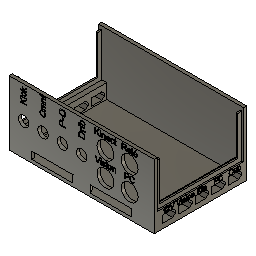
BlackBox+v3 (Autodesk Fusion 360 design; units mm, degrees)
Autodesk Fusion 360 part; units mm, degrees
(part 1 of 2)
sketch "Esboço1" plane through (0, 0, 0) normal (0, 1, 0) x (1, 0, 0)
  line L0 (0, 0) -> (0, -40)
  line L1 (90, 0) -> (-90, 0)
  line L2 (-90, 0) -> (-90, -80)
  line L3 (-90, -80) -> (90, -80)
  line L4 (90, -80) -> (90, 0)
  line L5 (90, 0) -> (-90, -80) construction
  line L6 (-90, 0) -> (90, -80) construction
  line L7 (90, -80) -> (70, -80)
  line L8 (70, -80) -> (70, -70)
  line L9 (70, -70) -> (90, -70)
  line L10 (90, -70) -> (90, -80)
  line L11 (70, -70) -> (49, -70)
  line L12 (49, -70) -> (49, -49)
  line L13 (49, -49) -> (70, -49)
  line L14 (70, -49) -> (70, -70)
  circle A0 centre (59.5, -59.5) radius 10.5
  circle A1 centre (29.5, -59.5) radius 10.5
  circle A2 centre (59.5, -29.5) radius 10.5
  circle A3 centre (29.5, -29.5) radius 10.5
  circle A4 centre (0, -40) radius 6.5
  line L15 (7.5, -24.75) -> (-7.5, -24.75)
  line L16 (-7.5, -24.75) -> (-7.5, -55.25)
  line L17 (-7.5, -55.25) -> (7.5, -55.25)
  line L18 (7.5, -55.25) -> (7.5, -24.75)
  line L19 (7.5, -24.75) -> (-7.5, -55.25) construction
  line L20 (-7.5, -24.75) -> (7.5, -55.25) construction
  line L21 (-31.5, -24.75) -> (-31.5, -55.25)
  line L22 (-31.5, -24.75) -> (-16.5, -55.25) construction
  line L23 (-16.5, -24.75) -> (-31.5, -55.25) construction
  line L24 (-31.5, -55.25) -> (-16.5, -55.25)
  circle A5 centre (-24, -40) radius 6.5
  line L25 (-16.5, -24.75) -> (-31.5, -24.75)
  line L26 (-16.5, -55.25) -> (-16.5, -24.75)
  line L27 (-55.5, -24.75) -> (-55.5, -55.25)
  line L28 (-55.5, -24.75) -> (-40.5, -55.25) construction
  line L29 (-40.5, -24.75) -> (-55.5, -55.25) construction
  line L30 (-55.5, -55.25) -> (-40.5, -55.25)
  circle A6 centre (-48, -40) radius 6.5
  line L31 (-40.5, -24.75) -> (-55.5, -24.75)
  line L32 (-40.5, -55.25) -> (-40.5, -24.75)
  line L33 (-79.5, -24.75) -> (-79.5, -55.25)
  line L34 (-79.5, -24.75) -> (-64.5, -55.25) construction
  line L35 (-64.5, -24.75) -> (-79.5, -55.25) construction
  line L36 (-79.5, -55.25) -> (-64.5, -55.25)
  circle A7 centre (-72, -40) radius 6.5
  line L37 (-64.5, -24.75) -> (-79.5, -24.75)
  line L38 (-64.5, -55.25) -> (-64.5, -24.75)
  line L39 (-86, -80) -> (-86, -4)
  line L40 (90, -80) -> (86, -80)
  line L41 (86, -80) -> (86, -4)
  line L42 (86, -4) -> (-86, -4)
  line L43 (11.25, -4) -> (11.25, -80)
  line L44 (15.25, -80) -> (15.25, -4)
  line L45 (15.25, -4) -> (11.25, -80) construction
  line L46 (11.25, -4) -> (15.25, -80) construction
  line L47 (-86, -4) -> (-62, -4)
  line L48 (-62, -4) -> (-7, -4)
  line L49 (-7, -4) -> (-7, -13)
  line L50 (-7, -13) -> (-62, -13)
  line L51 (-62, -13) -> (-62, -4)
  line L52 (86, -4) -> (62, -4)
  line L53 (62, -4) -> (7, -4)
  line L54 (7, -4) -> (7, -13)
  line L55 (7, -13) -> (62, -13)
  line L56 (62, -13) -> (62, -4)
  line L57 (86, -4) -> (86, -22)
  line L58 (86, -22) -> (90, -22)
  line L59 (-86, -4) -> (-86, -22)
  line L60 (-86, -22) -> (-90, -22)
  line L61 (-86, -4) -> (-90, -4)
  line L62 (86, -4) -> (90, -4)
  line L63 (29.5, -40) -> (29.5, -49)
  line L64 (39.5, -48.5) -> (19.5, -48.5)
  line L65 (19.5, -48.5) -> (19.5, -40.5)
  line L66 (19.5, -40.5) -> (39.5, -40.5)
  line L67 (39.5, -40.5) -> (39.5, -48.5)
  line L68 (39.5, -48.5) -> (19.5, -40.5) construction
  line L69 (19.5, -48.5) -> (39.5, -40.5) construction
  line L70 (19.5, -40.5) -> (39.5, -40.5) construction
  line L71 (39.5, -40.5) -> (39.5, -48.5) construction
  line L72 (39.5, -48.5) -> (19.5, -48.5) construction
  line L73 (19.5, -48.5) -> (19.5, -40.5) construction
  line L74 (19.5, -70.5) -> (39.5, -70.5) construction
  line L75 (39.5, -70.5) -> (39.5, -78.5) construction
  line L76 (39.5, -78.5) -> (19.5, -78.5) construction
  line L77 (19.5, -78.5) -> (19.5, -70.5) construction
  line L78 (49.5, -40.5) -> (69.5, -40.5) construction
  line L79 (69.5, -40.5) -> (69.5, -48.5) construction
  line L80 (69.5, -48.5) -> (49.5, -48.5) construction
  line L81 (49.5, -48.5) -> (49.5, -40.5) construction
  line L82 (49.5, -70.5) -> (69.5, -70.5) construction
  line L83 (69.5, -70.5) -> (69.5, -78.5) construction
  line L84 (69.5, -78.5) -> (49.5, -78.5) construction
  line L85 (49.5, -78.5) -> (49.5, -70.5) construction
  line L86 (4.0716, -57.4789) -> (4.0716, -77.4789) construction
  line L87 (4.0716, -77.4789) -> (-3.9284, -77.4789) construction
  line L88 (-3.9284, -77.4789) -> (-3.9284, -57.4789) construction
  line L89 (-3.9284, -57.4789) -> (4.0716, -57.4789) construction
  line L90 (-20.0052, -57.4897) -> (-20.0052, -77.4897) construction
  line L91 (-20.0052, -77.4897) -> (-28.0052, -77.4897) construction
  line L92 (-28.0052, -77.4897) -> (-28.0052, -57.4897) construction
  line L93 (-28.0052, -57.4897) -> (-20.0052, -57.4897) construction
  line L94 (-68.5263, -57.4789) -> (-68.5263, -77.4789) construction
  line L95 (-68.5263, -77.4789) -> (-76.5263, -77.4789) construction
  line L96 (-76.5263, -77.4789) -> (-76.5263, -57.4789) construction
  line L97 (-76.5263, -57.4789) -> (-68.5263, -57.4789) construction
  line L98 (-44.4564, -57.7899) -> (-44.5481, -77.8423) construction
  line L99 (-44.5481, -77.8423) -> (-52.4163, -77.8063) construction
  line L100 (-52.4163, -77.8063) -> (-52.3246, -57.7539) construction
  line L101 (-52.3246, -57.7539) -> (-44.4564, -57.7899) construction
  point P0 (0, -40)
  point P1 (0, -40)
  point P2 (-24, -40)
  point P3 (-24, -40)
  point P4 (-24, -40)
  point P5 (-48, -40)
  point P6 (-48, -40)
  point P7 (-48, -40)
  point P8 (-72, -40)
  point P9 (-72, -40)
  point P10 (-72, -40)
  point P11 (13.25, -42)
  point P12 (29.5, -44.5)
  dimension "d1" = 40
  dimension "d2" = 180
  dimension "d3" = 80
  dimension "d4" = 20
  dimension "d5" = 10
  dimension "d6" = 21
  dimension "d7" = 21
  dimension "d10" = -30
  dimension "d11" = 30
  dimension "d12" = 13
  dimension "d13" = 15
  dimension "d14" = 30.5
  dimension "d17" = -24
  dimension "d18" = 0
  dimension "d19" = 4
  dimension "d21" = 4
  dimension "d23" = 4
  dimension "d33" = 24
  dimension "d34" = 55
  dimension "d35" = 9
  dimension "d36" = 24
  dimension "d37" = 55
  dimension "d38" = 9
  dimension "d72" = 18
  dimension "d73" = 18
  dimension "d124" = 20
  dimension "d125" = 8
  dimension "d126" = 7
  dimension "d127" = 7
  dimension "d128" = 7
  dimension "d129" = 7
  dimension "d130" = 8
  dimension "d131" = 8
  dimension "d132" = 7
  dimension "d133" = 7
  text T0 "Vision" font "Arial" height 7 align centre middle in box 20 x 8 at (19.5, -40.5) x (1, 0) y (0, -1) spacing 1 kerned
  text T1 "Kinect" font "Arial" height 7 align centre middle in box 20 x 8 at (19.5, -70.5) x (1, 0) y (0, -1) spacing 1 kerned
  text T2 "PC" font "Arial" height 7 align centre middle in box 20 x 8 at (49.5, -40.5) x (1, 0) y (0, -1) spacing 1 kerned
  text T3 "Relé" font "Arial" height 7 align centre middle in box 20 x 8 at (49.5, -70.5) x (1, 0) y (0, -1) spacing 1 kerned
  text T4 "Drib" font "Arial" height 8 align centre middle in box 20 x 8 at (4.0716, -57.4789) x (0, -1) y (-1, 0) spacing 1 kerned
  text T5 "P-O" font "Arial" height 8 align centre middle in box 20 x 8 at (-20.0052, -57.4897) x (0, -1) y (-1, 0) spacing 1 kerned
  text T6 "Kick" font "Arial" height 7 align centre middle in box 20 x 8 at (-68.5263, -57.4789) x (0, -1) y (-1, 0) spacing 1 kerned
  text T7 "Omni" font "Arial" height 7 align centre middle in box 20.0526 x 7.8682 at (-44.4564, -57.7899) x (-0.004573, -0.99999) y (-0.99999, 0.004573) spacing 1 kerned
  constraint coincident L0.start origin
  constraint vertical L0
  constraint horizontal L1
  constraint parallel L2 L4
  constraint coincident L5 P1
  constraint coincident L6 P1
  constraint coincident P1 P0
  constraint horizontal L7
  constraint vertical L8
  constraint horizontal L9
  constraint vertical L10
  constraint horizontal L11
  constraint vertical L12
  constraint horizontal L13
  constraint vertical L14
  constraint tangent L11 A0
  constraint tangent L14 A0
  constraint tangent L13 A0
  constraint horizontal L15
  constraint perpendicular L15 L16
  constraint parallel L15 L17
  constraint parallel L16 L18
  constraint coincident L19 P1
  constraint coincident L20 P1
  constraint coincident L3 L39.start
  constraint coincident L7 L40.end
  constraint parallel L43 L44
  constraint coincident L45 P11
  constraint coincident L46 P11
  constraint coincident L42 L47.end
  constraint perpendicular L39 L47
  constraint horizontal L48
  constraint vertical L49
  constraint horizontal L50
  constraint vertical L51
  constraint coincident L42 L52.end
  constraint perpendicular L41 L52
  constraint horizontal L53
  constraint vertical L54
  constraint horizontal L55
  constraint vertical L56
  constraint coincident L41 L57.end
  constraint coincident L4 L58.end
  constraint perpendicular L4 L58
  constraint coincident L39 L59.end
  constraint coincident L2 L60.end
  constraint perpendicular L2 L60
  constraint coincident L2 L61.end
  constraint perpendicular L2 L61
  constraint coincident L4 L62.end
  constraint perpendicular L4 L62
  constraint coincident A3 L63.start
  constraint coincident A1 L63.end
  constraint vertical L63
  constraint horizontal L64
  constraint perpendicular L64 L65
  constraint parallel L64 L66
  constraint parallel L65 L67
  constraint coincident L68 P12
  constraint coincident L69 P12
  constraint midpoint L63 P12
  constraint coincident L66.end
  constraint coincident L64.end
  measures "d1" distance of L0.start P0
  measures "d2" distance of L2.end L3.end
  measures "d3" distance of L1.end L2.end
  measures "d4" distance of L3.end L7.end
  measures "d5" distance of L3.end L9.end
  measures "d6" distance of L8.end L11.end
  measures "d7" distance of L8.end L13.end
  measures "d12" diameter of A4
  measures "d13" distance of L16.end L17.end
  measures "d14" distance of L15.end L16.end
  measures "d19" distance of L2.end L39.start
  measures "d21" distance of L3.end L40.end
  measures "d23" distance of L43.end L44.start
  measures "d33" distance of L39.end L47.end
  measures "d34" distance of L47.end L48.end
  measures "d35" distance of L47.end L50.end
  measures "d36" distance of L41.end L52.end
  measures "d37" distance of L52.end L53.end
  measures "d38" distance of L52.end L55.end
  measures "d72" distance of L41.end L57.end
  measures "d73" distance of L39.end L59.end
  measures "d124" distance of L65.end L66.end
  measures "d125" distance of L64.end L65.end
sketch "Esboço3" plane through (0, 0, 0) normal (0, 0, 1) x (1, 0, 0)
  line L0 (90, 0) -> (-90, 0)
  line L1 (-90, 0) -> (90, 0)
  line L2 (90, 0) -> (90, 115)
  line L3 (90, 115) -> (-90, 115)
  line L4 (-90, 115) -> (-90, 0)
  point P0 (0, 55)
  point P1 (200, 0)
  point P2 (0, 55)
  point P3 (0, 55)
  point P4 (0, 55)
  dimension "d49" = 180
  dimension "d64" = 115
  constraint coincident P4 P3
  constraint horizontal L1
  constraint vertical L2
  constraint horizontal L3
  constraint vertical L4
  measures "d49" distance of L0.start L0.end
  measures "d64" distance of L0.end L3.end
extrude "Extrusão1" add sketch "Esboço1" along normal blind 4 contours L3 L39 L42 L43 L47 L49 L50 L51 L54 L55 L59 | L4 L41 L57 L58 L62 | L2 L39 L59 L60 L61 | L4 L9 L41 L58 | L11 L14 A0 | L3 L8 L9 L41 L42 L44 L52 L55 L56 L57 | L2 L3 L39 L60 | L3 L43 L44 L55 | L3 L4 L7 L9 L10 L40 L41 | L3 L7 L8 L9 L41 | L11 L12 A0 | L13 L14 A0 | L12 L13 A0 | L15 L16 L17 L18 | L21 L24 L25 L26 | L27 L30 L31 L32 | L33 L36 L37 L38 | L63 L64 L66 L67 | L63 L64 L65 L66 makes body 1
extrude "Extrusão2" add sketch "Esboço3" along normal blind 4 bodies 1
sketch "Esboço6" plane through (90, 0, 0) normal (1, 0, 0) x (0, 1, 0)
  line L0 (0, 0) -> (115, 0)
  line L1 (115, 0) -> (115, 4)
  line L2 (115, 4) -> (4, 4)
  line L3 (0, 80) -> (0, 0)
  line L4 (0, 4) -> (10, 4)
  line L5 (10, 4) -> (10, 6)
  line L6 (10, 15) -> (23, 15)
  line L7 (23, 15) -> (26.5, 12)
  line L8 (26.5, 12) -> (26.5, 9)
  line L9 (23, 6) -> (26.5, 9)
  line L10 (10, 6) -> (23, 6)
  line L11 (10, 15) -> (10, 6)
  line L12 (43.5, 15) -> (47, 12)
  line L13 (30.5, 15) -> (43.5, 15)
  line L14 (30.5, 15) -> (30.5, 6)
  line L15 (30.5, 6) -> (43.5, 6)
  line L16 (43.5, 6) -> (47, 9)
  line L17 (47, 12) -> (47, 9)
  line L18 (64, 15) -> (67.5, 12)
  line L19 (51, 15) -> (64, 15)
  line L20 (51, 15) -> (51, 6)
  line L21 (51, 6) -> (64, 6)
  line L22 (64, 6) -> (67.5, 9)
  line L23 (67.5, 12) -> (67.5, 9)
  line L24 (84.5, 15) -> (88, 12)
  line L25 (71.5, 15) -> (84.5, 15)
  line L26 (71.5, 15) -> (71.5, 6)
  line L27 (71.5, 6) -> (84.5, 6)
  line L28 (84.5, 6) -> (88, 9)
  line L29 (88, 12) -> (88, 9)
  line L30 (105, 15) -> (108.5, 12)
  line L31 (92, 15) -> (105, 15)
  line L32 (92, 15) -> (92, 6)
  line L33 (92, 6) -> (105, 6)
  line L34 (105, 6) -> (108.5, 9)
  line L35 (108.5, 12) -> (108.5, 9)
  line L36 (115, 4) -> (111, 4)
  line L37 (0, 4) -> (0, 22)
  line L38 (0, 22) -> (115, 22)
  line L39 (115, 22) -> (115, 4)
  line L40 (0, 4) -> (4, 4)
  line L41 (4, 4) -> (4, 22)
  line L42 (4, 22) -> (0, 22)
  line L43 (0, 22) -> (0, 4)
  line L44 (4, 4) -> (4, 80)
  line L45 (105, 15) -> (108.5, 12)
  line L46 (30.5, 6) -> (43.5, 6)
  line L47 (0, 22) -> (115, 22)
  line L48 (30.5, 15) -> (43.5, 15)
  line L49 (92, 15) -> (105, 15)
  line L50 (23, 6) -> (26.5, 9)
  line L51 (108.5, 12) -> (108.5, 9)
  line L52 (115, 4) -> (4, 4)
  line L53 (10, 15) -> (10, 6)
  line L54 (43.5, 15) -> (47, 12)
  line L55 (0, 4) -> (10, 4)
  line L56 (0, 4) -> (0, 22)
  line L57 (10, 6) -> (23, 6)
  line L58 (0, 22) -> (0, 0)
  line L59 (67.5, 12) -> (67.5, 9)
  line L60 (64, 6) -> (67.5, 9)
  line L61 (84.5, 15) -> (88, 12)
  line L62 (10, 15) -> (23, 15)
  line L63 (26.5, 12) -> (26.5, 9)
  line L64 (0, 0) -> (115, 0)
  line L65 (115, 0) -> (115, 4)
  line L66 (71.5, 15) -> (84.5, 15)
  line L67 (92, 15) -> (92, 6)
  line L68 (88, 12) -> (88, 9)
  line L69 (115, 4) -> (111, 4)
  line L70 (71.5, 6) -> (84.5, 6)
  line L71 (115, 22) -> (115, 4)
  line L72 (92, 6) -> (105, 6)
  line L73 (51, 6) -> (64, 6)
  line L74 (105, 6) -> (108.5, 9)
  line L75 (64, 15) -> (67.5, 12)
  line L76 (10, 4) -> (10, 6)
  line L77 (71.5, 15) -> (71.5, 6)
  line L78 (0, 4) -> (4, 4)
  line L79 (4, 4) -> (4, 22)
  line L80 (0, 22) -> (0, 4)
  line L81 (4, 4) -> (4, 22)
  line L82 (23, 15) -> (26.5, 12)
  line L83 (47, 12) -> (47, 9)
  line L84 (4, 22) -> (0, 22)
  line L85 (30.5, 15) -> (30.5, 6)
  line L86 (84.5, 6) -> (88, 9)
  line L87 (51, 15) -> (51, 6)
  line L88 (51, 15) -> (64, 15)
  line L89 (43.5, 6) -> (47, 9)
  line L90 (4, 22) -> (0, 22)
  line L91 (4, 80) -> (0, 80)
  line L92 (10, 15) -> (26.5, 15)
  line L93 (26.5, 15) -> (26.5, 22)
  line L94 (26.5, 22) -> (10, 22)
  line L95 (10, 22) -> (10, 15)
  line L96 (10, 15) -> (26.5, 15) construction
  line L97 (26.5, 15) -> (26.5, 22) construction
  line L98 (26.5, 22) -> (10, 22) construction
  line L99 (10, 22) -> (10, 15) construction
  line L100 (30.5, 15) -> (47, 15) construction
  line L101 (47, 15) -> (47, 22) construction
  line L102 (47, 22) -> (30.5, 22) construction
  line L103 (30.5, 22) -> (30.5, 15) construction
  line L104 (51, 15) -> (67.5, 15) construction
  line L105 (67.5, 15) -> (67.5, 22) construction
  line L106 (67.5, 22) -> (51, 22) construction
  line L107 (51, 22) -> (51, 15) construction
  line L108 (71.5, 15) -> (88, 15) construction
  line L109 (88, 15) -> (88, 22) construction
  line L110 (88, 22) -> (71.5, 22) construction
  line L111 (71.5, 22) -> (71.5, 15) construction
  line L112 (92, 15) -> (108.5, 15) construction
  line L113 (108.5, 15) -> (108.5, 22) construction
  line L114 (108.5, 22) -> (92, 22) construction
  line L115 (92, 22) -> (92, 15) construction
  dimension "d65" = 10
  dimension "d66" = 2
  dimension "d69" = 20.5
  dimension "d70" = 0
  dimension "d71" = 4
  dimension "d77" = 4
  dimension "d82" = 20.5
  dimension "d83" = 0
  dimension "d84" = 10
  dimension "d85" = 2
  dimension "d86" = 4
  dimension "d87" = 4
  dimension "d136" = 6
  dimension "d137" = 6
  dimension "d138" = 6
  dimension "d139" = 6
  dimension "d140" = 6
  text T0 "12V" font "Arial" height 6 align centre middle in box 16.5 x 7 at (10, 15) x (1, 0) y (0, 1) spacing 1 kerned
  text T1 "Vision" font "Arial" height 6 align centre middle in box 16.5 x 7 at (30.5, 15) x (1, 0) y (0, 1) spacing 1 kerned
  text T2 "Kin" font "Arial" height 6 align centre middle in box 16.5 x 7 at (51, 15) x (1, 0) y (0, 1) spacing 1 kerned
  text T3 "PC" font "Arial" height 6 align centre middle in box 16.5 x 7 at (71.5, 15) x (1, 0) y (0, 1) spacing 1 kerned
  text T4 "Cap" font "Arial" height 6 align centre middle in box 16.5 x 7 at (92, 15) x (1, 0) y (0, 1) spacing 1 kerned
  constraint perpendicular L4 L5
  constraint vertical L11
  constraint perpendicular L6 L11
  constraint perpendicular L10 L11
  constraint coincident L1.end L2.start
  constraint coincident L2 L36.end
  constraint perpendicular L4 L37
  constraint perpendicular L1 L38
  constraint perpendicular L2 L39
  constraint horizontal L40
  constraint vertical L41
  constraint horizontal L42
  constraint vertical L43
  constraint perpendicular L55 L76
  constraint vertical L53
  constraint perpendicular L53 L62
  constraint perpendicular L53 L57
  constraint coincident L36.end L52
  constraint perpendicular L55 L56
  constraint perpendicular L47 L65
  constraint perpendicular L52 L71
  constraint horizontal L78
  constraint vertical L79
  constraint horizontal L84
  constraint vertical L80
  constraint horizontal L92
  constraint vertical L93
  constraint horizontal L94
  constraint vertical L95
  constraint coincident L38 L93.end
  constraint coincident L92.end
  constraint coincident L94.end
  measures "d65" distance of L4.start L4.end
  measures "d66" distance of L5.end L4.end
  measures "d71" distance of L1.end L36.end
  measures "d77" distance of L4.start L2.end
  measures "d84" distance of L4.end L4.start
  measures "d85" distance of L4.end L5.end
  measures "d86" distance of L1.end L36.end
  measures "d87" distance of L4.start L2.end
extrude "Extrusão3" add sketch "Esboço6" against normal blind 10 contours L2 L5 L7 L8 L9 L10 L36 L38 L39 L47 L50 L52 L57 L63 L69 L71 L76 L82 L92 L93 | L2 L4 L5 L11 L38 L41 L44 L47 L52 L53 L55 L76 L79 L81 L95 | L6 L38 L47 L62 L92 L93 L94 L95 bodies 1
sketch "Esboço7" plane through (-90, 0, 0) normal (-1, 0, 0) x (0, -1, 0)
  line L0 (0, 0) -> (0, 80)
  line L1 (-4, 80) -> (-4, 4)
  line L2 (-4, 4) -> (-115, 4)
  line L3 (-115, 4) -> (-115, 0)
  line L4 (-115, 0) -> (0, 0)
  line L5 (-4, 4) -> (-4, 6)
  line L6 (-4, 6) -> (-10, 6)
  line L7 (-26.5, 9) -> (-26.5, 12)
  line L8 (-23, 15) -> (-26.5, 12)
  line L9 (-23, 15) -> (-26.5, 12)
  line L10 (-10, 6) -> (-10, 15)
  line L11 (-23, 6) -> (-26.5, 9)
  line L12 (-23, 6) -> (-26.5, 9)
  line L13 (-26.5, 9) -> (-26.5, 12)
  line L14 (-10, 15) -> (-23, 15)
  line L15 (-10, 6) -> (-23, 6)
  line L16 (-10, 15) -> (-23, 15)
  line L17 (-10, 6) -> (-23, 6)
  line L18 (-10, 6) -> (-10, 15)
  line L19 (-30.5, 6) -> (-43.5, 6)
  line L20 (-43.5, 6) -> (-47, 9)
  line L21 (-47, 9) -> (-47, 12)
  line L22 (-43.5, 15) -> (-47, 12)
  line L23 (-30.5, 15) -> (-43.5, 15)
  line L24 (-30.5, 6) -> (-30.5, 15)
  line L25 (-51, 6) -> (-64, 6)
  line L26 (-64, 6) -> (-67.5, 9)
  line L27 (-67.5, 9) -> (-67.5, 12)
  line L28 (-64, 15) -> (-67.5, 12)
  line L29 (-51, 15) -> (-64, 15)
  line L30 (-51, 6) -> (-51, 15)
  line L31 (-71.5, 6) -> (-84.5, 6)
  line L32 (-84.5, 6) -> (-88, 9)
  line L33 (-88, 9) -> (-88, 12)
  line L34 (-84.5, 15) -> (-88, 12)
  line L35 (-71.5, 15) -> (-84.5, 15)
  line L36 (-71.5, 6) -> (-71.5, 15)
  line L37 (-92, 6) -> (-105, 6)
  line L38 (-105, 6) -> (-108.5, 9)
  line L39 (-108.5, 9) -> (-108.5, 12)
  line L40 (-105, 15) -> (-108.5, 12)
  line L41 (-92, 15) -> (-105, 15)
  line L42 (-92, 6) -> (-92, 15)
  line L43 (0, 4) -> (-115, 4)
  line L44 (-115, 4) -> (-115, 22)
  line L45 (-115, 22) -> (0, 22)
  line L46 (0, 22) -> (0, 4)
  line L47 (0, 80) -> (-4, 80)
  line L48 (-10, 15) -> (-26.5, 15)
  line L49 (-26.5, 15) -> (-26.5, 22)
  line L50 (-26.5, 22) -> (-10, 22)
  line L51 (-10, 22) -> (-10, 15)
  line L52 (-26.5, 15) -> (-10, 15) construction
  line L53 (-10, 15) -> (-10, 22) construction
  line L54 (-10, 22) -> (-26.5, 22) construction
  line L55 (-26.5, 22) -> (-26.5, 15) construction
  line L56 (-47, 15) -> (-30.5, 15) construction
  line L57 (-30.5, 15) -> (-30.5, 22) construction
  line L58 (-30.5, 22) -> (-47, 22) construction
  line L59 (-47, 22) -> (-47, 15) construction
  line L60 (-67.5, 15) -> (-51, 15) construction
  line L61 (-51, 15) -> (-51, 22) construction
  line L62 (-51, 22) -> (-67.5, 22) construction
  line L63 (-67.5, 22) -> (-67.5, 15) construction
  line L64 (-88, 15) -> (-71.5, 15) construction
  line L65 (-71.5, 15) -> (-71.5, 22) construction
  line L66 (-71.5, 22) -> (-88, 22) construction
  line L67 (-88, 22) -> (-88, 15) construction
  line L68 (-108.5, 15) -> (-92, 15) construction
  line L69 (-92, 15) -> (-92, 22) construction
  line L70 (-92, 22) -> (-108.5, 22) construction
  line L71 (-108.5, 22) -> (-108.5, 15) construction
  dimension "d88" = 2
  dimension "d89" = 6
  dimension "d92" = -20.5
  dimension "d93" = 0
  dimension "d99" = 115
  dimension "d100" = 18
  dimension "d143" = 6
  dimension "d144" = 6
  dimension "d145" = 6
  dimension "d146" = 6
  dimension "d147" = 6
  text T0 "Kick" font "Arial" height 6 align centre middle in box 16.5 x 7 at (-26.5, 15) x (1, 0) y (0, 1) spacing 1 kerned
  text T1 "Omni" font "Arial" height 6 align centre middle in box 16.5 x 7 at (-47, 15) x (1, 0) y (0, 1) spacing 1 kerned
  text T2 "P-O" font "Arial" height 6 align centre middle in box 16.5 x 7 at (-67.5, 15) x (1, 0) y (0, 1) spacing 1 kerned
  text T3 "Drib" font "Arial" height 6 align centre middle in box 16.5 x 7 at (-88, 15) x (1, 0) y (0, 1) spacing 1 kerned
  text T4 "24V" font "Arial" height 6 align centre middle in box 16.5 x 7 at (-108.5, 15) x (1, 0) y (0, 1) spacing 1 kerned
  constraint coincident L1.end L2.start
  constraint coincident L1 L5.end
  constraint perpendicular L5 L6
  constraint horizontal L43
  constraint vertical L44
  constraint horizontal L45
  constraint vertical L46
  constraint coincident L0 L43.start
  constraint horizontal L48
  constraint vertical L49
  constraint horizontal L50
  constraint vertical L51
  constraint coincident L45 L49.end
  constraint coincident L49.end
  constraint coincident L10.end
  measures "d88" distance of L1.end L5.end
  measures "d89" distance of L5.end L6.end
  measures "d99" distance of L43.start L2.end
  measures "d100" distance of L43.start L45.end
extrude "Extrusão4" add sketch "Esboço7" against normal blind 10 contours L1 L2 L5 L6 L7 L8 L9 L11 L12 L13 L15 L17 L43 L44 L45 L48 L49 | L1 L6 L10 L18 L45 L51 | L14 L16 L45 L48 L49 L50 L51 bodies 1
sketch "Esboço8" plane through (0, 0, 4) normal (0, 0, 1) x (-1, 0, 0)
  line L0 (80, -115) -> (80, -4)
  line L1 (80, -4) -> (62, -4)
  line L2 (62, -4) -> (62, 0)
  line L3 (62, 0) -> (7, 0)
  line L4 (7, 0) -> (7, -4)
  line L5 (7, -4) -> (-7, -4)
  line L6 (-7, -4) -> (-7, 0)
  line L7 (-7, 0) -> (-62, 0)
  line L8 (-62, 0) -> (-62, -4)
  line L9 (-62, -4) -> (-80, -4)
  line L10 (-80, -4) -> (-80, -115)
  line L11 (-80, -115) -> (80, -115)
  line L12 (7, 0) -> (11, 0)
  line L13 (7, 0) -> (7, -7)
  line L14 (7, -7) -> (11, 0)
  line L15 (-7, 0) -> (-11, 0)
  line L16 (-7, 0) -> (-7, -7)
  line L17 (-7, -7) -> (-11, 0)
  line L18 (-7, -4) -> (7, -4)
  line L19 (7, -4) -> (7, -7)
  line L20 (7, -7) -> (-7, -7)
  line L21 (-7, -7) -> (-7, -4)
  dimension "d101" = 4
  dimension "d102" = 7
  dimension "d103" = 4
  dimension "d104" = 7
  constraint coincident L3.end L4.start
  constraint perpendicular L4 L12
  constraint perpendicular L12 L13
  constraint coincident L6.end L7.start
  constraint perpendicular L6 L15
  constraint perpendicular L15 L16
  constraint horizontal L18
  constraint vertical L19
  constraint horizontal L20
  constraint vertical L21
  constraint coincident L5.end L6.start
  measures "d101" distance of L3.end L12.end
  measures "d102" distance of L3.end L13.end
  measures "d103" distance of L6.end L15.end
  measures "d104" distance of L6.end L16.end
extrude "Extrusão5" add sketch "Esboço8" along normal blind 9 contours L3 L4 L12 L13 L14 L19 | L5 L13 L16 L18 L19 L20 L21 | L6 L7 L15 L16 L17 L21 bodies 1
sketch "Esboço10" plane through (0, 115, 0) normal (0, 1, 0) x (-1, 0, 0)
  line L0 (-90, 0) -> (90, 0)
  line L1 (90, 0) -> (90, 22)
  line L2 (90, 22) -> (80, 22)
  line L3 (80, 22) -> (80, 4)
  line L4 (80, 4) -> (-80, 4)
  line L5 (-80, 4) -> (-80, 22)
  line L6 (-80, 22) -> (-90, 22)
  line L7 (-90, 22) -> (-90, 0)
  line L8 (-90, 0) -> (90, 0)
  line L9 (90, 0) -> (90, 80)
  line L10 (90, 80) -> (-90, 80)
  line L11 (-90, 80) -> (-90, 0)
  line L12 (-90, 22) -> (-88, 22)
  line L13 (-88, 22) -> (-88, 27)
  line L14 (-88, 27) -> (-86, 27)
  line L15 (-86, 27) -> (-86, 22)
  line L16 (-88, 27) -> (-86, 27)
  line L17 (-86, 27) -> (-86, 80)
  line L18 (-86, 80) -> (-88, 80)
  line L19 (-88, 80) -> (-88, 27)
  line L20 (90, 22) -> (88, 22)
  line L21 (88, 22) -> (88, 27)
  line L22 (88, 27) -> (86, 27)
  line L23 (86, 27) -> (86, 22)
  line L24 (88, 27) -> (86, 27)
  line L25 (86, 27) -> (86, 80)
  line L26 (86, 80) -> (88, 80)
  line L27 (88, 80) -> (88, 27)
  line L28 (-88, 80) -> (-86, 80)
  line L29 (-86, 80) -> (-86, 75.5)
  line L30 (-86, 75.5) -> (-88, 75.5)
  line L31 (-88, 75.5) -> (-88, 80)
  line L32 (86, 80) -> (88, 80)
  line L33 (88, 80) -> (88, 75.5)
  line L34 (88, 75.5) -> (86, 75.5)
  line L35 (86, 75.5) -> (86, 80)
  dimension "d107" = 80
  dimension "d108" = 2
  dimension "d109" = 5
  dimension "d110" = 2
  dimension "d111" = 2
  dimension "d112" = 5
  dimension "d113" = 2
  dimension "d114" = 5
  dimension "d152" = 4.5
  dimension "d153" = 4.5
  constraint horizontal L8
  constraint vertical L9
  constraint horizontal L10
  constraint vertical L11
  constraint coincident L0.start L7.end
  constraint coincident L6.end L7.start
  constraint coincident L6 L12.end
  constraint perpendicular L12 L13
  constraint perpendicular L13 L14
  constraint coincident L6 L15.end
  constraint perpendicular L6 L15
  constraint horizontal L16
  constraint vertical L17
  constraint horizontal L18
  constraint vertical L19
  constraint coincident L10 L17.end
  constraint coincident L1.end L2.start
  constraint perpendicular L9 L20
  constraint perpendicular L20 L21
  constraint perpendicular L21 L22
  constraint perpendicular L2 L23
  constraint horizontal L24
  constraint vertical L25
  constraint horizontal L26
  constraint vertical L27
  constraint coincident L10 L25.end
  constraint horizontal L28
  constraint vertical L29
  constraint horizontal L30
  constraint vertical L31
  constraint horizontal L32
  constraint vertical L33
  constraint horizontal L34
  constraint vertical L35
  measures "d107" distance of L0.start L10.end
  measures "d108" distance of L6.end L12.end
  measures "d109" distance of L12.end L13.end
  measures "d110" distance of L13.end L14.end
  measures "d111" distance of L1.end L20.end
  measures "d112" distance of L20.end L21.end
  measures "d113" distance of L21.end L22.end
  measures "d114" distance of L22.end L23.end
  measures "d152" distance of L18.end L30.end
  measures "d153" distance of L25.end L34.end
extrude "Extrusão6" add sketch "Esboço10" against normal blind 9 separate body contours L14 L16 L17 L19 L30 | L22 L24 L25 L27 L34 makes body 2 at (-86, 112, 43.1667) makes body 3 at (88, 112, 59.3333)
extrude "Extrusão7" add sketch "Esboço10" against normal blind 115 contours L6 L13 L14 L15 L16 | L2 L21 L22 L23 L24 bodies 1 2 3
extrude "Extrusão8" add sketch "Esboço10" along normal blind 5 from surface at -111 contours L14 L16 L17 L19 L30 | L22 L24 L25 L27 L34 bodies 1
extrude "Extrusão9" add sketch "Esboço10" against normal blind 4 contours L6 L10 L11 L12 L13 L19 L31 | L2 L9 L10 L20 L21 L27 L33 | L2 L3 L4 L5 L6 L10 L15 L17 L23 L25 L29 L35 | L10 L17 L18 L19 L28 L29 L30 L31 | L10 L25 L26 L27 L32 L33 L34 L35 bodies 1
extrude "Extrusão10" cut sketch "Esboço1" along normal blind 1 text T6 T7 T5 T4 T1 T3 T2 T0 bodies 1
extrude "Extrusão12" cut sketch "Esboço7" against normal blind 1 text T1 T2 T3 T4 T0 bodies 1
extrude "Extrusão13" cut sketch "Esboço6" against normal blind 1 text T4 T3 T2 T1 T0 bodies 1
sketch "Esboço11" plane through (0, 0, 80) normal (0, 0, 1) x (-1, 0, 0)
  line L0 (90, 0) -> (-90, 0)
  line L1 (-90, 0) -> (-90, -4)
  line L2 (-90, -4) -> (90, -4)
  line L3 (90, -4) -> (90, 0)
  line L4 (-90, 0) -> (90, 0)
  line L5 (90, 0) -> (90, -115)
  line L6 (90, -115) -> (-90, -115)
  line L7 (-90, -115) -> (-90, 0)
  line L8 (-90, -115) -> (90, -115)
  line L9 (90, -115) -> (90, -111)
  line L10 (90, -111) -> (-90, -111)
  line L11 (-90, -111) -> (-90, -115)
  line L12 (90, -111) -> (88.5, -111)
  line L13 (88.5, -111) -> (88.5, -105.5)
  line L14 (88.5, -105.5) -> (85.5, -105.5)
  line L15 (85.5, -105.5) -> (85.5, -111)
  line L16 (85.5, -111) -> (84, -111)
  line L17 (84, -111) -> (84, -4)
  line L18 (90, -4) -> (88.5, -4)
  line L19 (88.5, -4) -> (88.5, -9.5)
  line L20 (88.5, -9.5) -> (85.5, -9.5)
  line L21 (85.5, -9.5) -> (85.5, -4)
  line L22 (84, -4) -> (85.5, -4)
  line L23 (0, -2.5) -> (0, -20)
  line L24 (-84, -111) -> (-84, -4)
  line L25 (-85.5, -111) -> (-84, -111)
  line L26 (-85.5, -105.5) -> (-85.5, -111)
  line L27 (-88.5, -105.5) -> (-85.5, -105.5)
  line L28 (-88.5, -111) -> (-88.5, -105.5)
  line L29 (-90, -4) -> (-88.5, -4)
  line L30 (-88.5, -4) -> (-88.5, -9.5)
  line L31 (-88.5, -9.5) -> (-85.5, -9.5)
  line L32 (-85.5, -9.5) -> (-85.5, -4)
  line L33 (-84, -4) -> (-85.5, -4)
  spline S0 degree 2 poles (-63.8808, -17.9485) (-63.4219, -17.7584) (-62.682, -17.7569) knots 0 0 0 1 1 1
  line L34 (-70.8016, -23.1354) -> (-67.3955, -18.923)
  line L35 (38.4038, -69.3744) -> (40.6197, -69.3744)
  circle A0 centre (39.0194, -15.5804) radius 1.0182
  line L36 (-42.4097, -22.7295) -> (-42.4196, -17.8223)
  spline S1 degree 2 poles (-37.515, -20.772) (-37.5173, -19.6494) (-37.4162, -19.1857) knots 0 0 0 1 1 1
  spline S2 degree 5 poles (37.5794, -16.5404) (37.5731, -16.5497) (37.56, -16.5673) (37.538, -16.5913) (37.5043, -16.6183) (37.4543, -16.6431) (37.3957, -16.6583) (37.328, -16.6632) (37.251, -16.6575) (37.165, -16.6417) (37.071, -16.6168) (36.9898, -16.5902) (36.9258, -16.5666) (36.8817, -16.5494) (36.8594, -16.5404) knots 0 0 0 0 0 0 0.1 0.2 0.3 0.4 0.5 0.6 0.7 0.8 0.9 1 1 1 1 1 1
  line L37 (61.9394, -28.4241) -> (62.5394, -26.1404)
  arc A1 (43.4662, -59.2854) -> (42.4188, -59.63) centre (42.9425, -59.4577) ccw
  line L38 (-50.1198, -20.3042) -> (-51.8207, -20.3076)
  spline S3 degree 5 poles (59.4686, -20.1404) (59.4344, -20.1707) (59.3633, -20.2283) (59.2486, -20.3057) (59.0795, -20.3909) (58.841, -20.4666) (58.5758, -20.5103) (58.2857, -20.5213) (57.9752, -20.4992) (57.6509, -20.4444) (57.3208, -20.3574) (56.9927, -20.2392) (56.6739, -20.0909) (56.3697, -19.9139) (56.0828, -19.7097) (55.8146, -19.4796) (55.6152, -19.2759) (55.474, -19.1123) (55.3836, -18.9985) (55.3394, -18.9404) knots 0 0 0 0 0 0 0.066667 0.133333 0.2 0.266667 0.333333 0.4 0.466667 0.533333 0.6 0.666667 0.733333 0.8 0.866667 0.933333 1 1 1 1 1 1
  line L39 (37.8194, -14.5004) -> (37.0994, -14.5004)
  line L40 (-20.2167, -16.7211) -> (-20.2167, -16.3211)
  spline S4 degree 2 poles (-37.0414, -18.4025) (-36.7678, -18.0831) (-36.3089, -17.8929) knots 0 0 0 1 1 1
  line L41 (45.922, -17.1567) -> (44.5601, -22.3879)
  line L42 (56.6139, -18.0567) -> (55.3394, -18.9404)
  line L43 (-17.5602, -15.6077) -> (-19.9792, -16.8211)
  line L44 (-41.2503, -17.82) -> (-41.2377, -24.0538)
  line L45 (-17.0167, -17.5348) -> (-20.4792, -17.5348)
  line L46 (43.3064, -15.6436) -> (43.5442, -14.4114)
  arc A2 (37.9455, -63.0285) -> (38.7844, -62.562) centre (38.365, -62.7953) ccw
  arc A3 (38.4038, -68.2176) -> (38.4038, -69.3744) centre (38.4038, -68.796) ccw
  line L47 (-20.4792, -17.5348) -> (-20.4792, -16.7211)
  spline S5 degree 2 poles (-36.3089, -17.8929) (-35.8501, -17.7028) (-35.1102, -17.7013) knots 0 0 0 1 1 1
  line L48 (40.6197, -68.2176) -> (38.4038, -68.2176)
  line L49 (-36.2567, -20.5952) -> (-36.2497, -24.0438)
  line L50 (-20.2167, -16.3211) -> (-20.4792, -16.3211)
  arc A4 (48.9725, -70.3446) -> (48.9725, -71.6116) centre (48.9725, -70.9781) ccw
  line L51 (40.6197, -68.796) -> (38.4038, -68.796) construction
  spline S6 degree 5 poles (37.3394, -16.0604) (37.3406, -16.0739) (37.3433, -16.1006) (37.3483, -16.1396) (37.3569, -16.1896) (37.3711, -16.2483) (37.3889, -16.303) (37.4108, -16.3533) (37.4368, -16.3991) (37.4669, -16.4405) (37.5008, -16.4777) (37.5306, -16.5046) (37.5544, -16.5231) (37.571, -16.5348) (37.5794, -16.5404) knots 0 0 0 0 0 0 0.1 0.2 0.3 0.4 0.5 0.6 0.7 0.8 0.9 1 1 1 1 1 1
  line L52 (61.8287, -14.4338) -> (60.1394, -14.4338)
  line L53 (63.4985, -28.4241) -> (65.3521, -22.4047)
  line L54 (-47.2715, -17.8321) -> (-46.1021, -17.8298)
  spline S7 degree 5 poles (61.3394, -20.1404) (61.3113, -20.1689) (61.2542, -20.2234) (61.1662, -20.2975) (61.0437, -20.3809) (60.8817, -20.4577) (60.71, -20.5048) (60.5279, -20.52) (60.3351, -20.5025) (60.1322, -20.4539) (59.92, -20.3769) (59.7434, -20.2944) (59.6074, -20.2216) (59.5152, -20.1683) (59.4686, -20.1404) knots 0 0 0 0 0 0 0.1 0.2 0.3 0.4 0.5 0.6 0.7 0.8 0.9 1 1 1 1 1 1
  line L55 (45.6038, -61.9232) -> (48.765, -61.9232)
  line L56 (41.6483, -24.5507) -> (42.4644, -27.5429)
  line L57 (34.1976, -14.3804) -> (33.4994, -14.3804)
  line L58 (33.4994, -14.3804) -> (33.2812, -15.5804)
  spline S8 degree 2 poles (-16.8448, -26.5035) (-17.1159, -27.0086) (-17.6398, -27.279) knots 0 0 0 1 1 1
  line L59 (36.0194, -14.3804) -> (35.2994, -14.3804)
  line L60 (-38.8094, -17.815) -> (-38.7969, -24.0489)
  spline S9 degree 2 poles (-19.2415, -26.5948) (-18.9988, -26.7715) (-18.6359, -26.7707) knots 0 0 0 1 1 1
  line L61 (39.9627, -59.5046) -> (39.9627, -66.5435)
  line L62 (42.7329, -22.3879) -> (44.3007, -16.8973)
  line L63 (-51.8207, -20.3076) -> (-50.9571, -22.6191)
  line L64 (36.0527, -59.6242) -> (37.9455, -63.0285)
  line L65 (-42.4196, -17.8223) -> (-41.2503, -17.82)
  spline S10 degree 2 poles (-61.3273, -17.9604) (-60.8655, -18.1657) (-60.5969, -18.4947) knots 0 0 0 1 1 1
  line L66 (-37.5084, -24.0463) -> (-37.515, -20.772)
  spline S11 degree 2 poles (-18.6332, -23.9075) (-18.8968, -23.908) (-19.1617, -24.012) knots 0 0 0 1 1 1
  line L67 (-56.1014, -18.9002) -> (-59.2311, -18.9066)
  spline S12 degree 5 poles (62.5394, -26.1404) (62.479, -26.1137) (62.3563, -26.0624) (62.1669, -25.9924) (61.9035, -25.9127) (61.5572, -25.833) (61.1971, -25.7636) (60.83, -25.6862) (60.4679, -25.5675) (60.1273, -25.3662) (59.8284, -25.0483) (59.5939, -24.6017) (59.4473, -24.0492) (59.4131, -23.4699) (59.4929, -22.9099) (59.675, -22.3991) (59.9384, -21.9511) (60.2583, -21.5702) (60.6109, -21.2543) (60.9793, -21.0003) (61.354, -20.8057) (61.7301, -20.668) (62.1059, -20.5847) (62.4807, -20.5538) (62.8525, -20.5734) (63.2184, -20.6419) (63.5747, -20.7579) (63.9175, -20.9202) (64.2439, -21.1276) (64.5519, -21.3794) (64.8403, -21.6747) (65.055, -21.9454) (65.207, -22.1676) (65.3044, -22.3242) (65.3521, -22.4047) knots 0 0 0 0 0 0 0.033333 0.066667 0.1 0.133333 0.166667 0.2 0.233333 0.266667 0.3 0.333333 0.366667 0.4 0.433333 0.466667 0.5 0.533333 0.566667 0.6 0.633333 0.666667 0.7 0.733333 0.766667 0.8 0.833333 0.866667 0.9 0.933333 0.966667 1 1 1 1 1 1
  line L68 (59.8105, -25.3318) -> (59.2683, -23.3491)
  spline S13 degree 2 poles (-60.2426, -19.185) (-60.1182, -19.7205) (-60.1161, -20.7666) knots 0 0 0 1 1 1
  line L69 (-40.0555, -24.0514) -> (-40.0681, -17.8176)
  line L70 (63.4985, -28.4241) -> (61.9394, -28.4241)
  arc A5 (48.765, -61.9232) -> (48.765, -60.4176) centre (48.765, -61.1704) ccw
  line L71 (37.0994, -14.5004) -> (36.7044, -15.7841)
  line L72 (-40.0681, -17.8176) -> (-38.8094, -17.815)
  line L73 (45.3123, -66.6609) -> (42.9425, -59.4577) construction
  line L74 (-46.1021, -17.8298) -> (-46.0922, -22.7369)
  line L75 (-19.9784, -17.1404) -> (-19.0773, -17.1386)
  arc A6 (39.9627, -66.5435) -> (41.2766, -66.5435) centre (40.6197, -66.5435) ccw
  line L76 (48.9725, -71.6116) -> (55.6595, -71.6116)
  line L77 (-19.0773, -17.1386) -> (-17.5602, -16.3775)
  arc A7 (38.4093, -62.7955) -> (36.5938, -67.6359) centre (38.3745, -65.5431) ccw construction
  line L78 (38.7844, -62.562) -> (36.8916, -59.1577)
  line L79 (40.6992, -15.1826) -> (40.3652, -14.7618)
  line L80 (48.765, -60.4176) -> (45.6038, -60.4176)
  spline S14 degree 5 poles (35.0594, -15.5804) (35.0581, -15.5839) (35.0537, -15.5918) (35.0421, -15.6069) (35.0164, -15.6335) (34.967, -15.6772) (34.9013, -15.7303) (34.8206, -15.7909) (34.7281, -15.8549) (34.6286, -15.9164) (34.5277, -15.9688) (34.4312, -16.0053) (34.3443, -16.0208) (34.2705, -16.0125) (34.211, -15.9813) (34.1645, -15.9319) (34.1285, -15.8708) (34.0995, -15.8053) (34.0745, -15.7421) (34.051, -15.6858) (34.0277, -15.639) (34.0087, -15.6101) (33.9942, -15.5934) (33.9843, -15.5844) (33.9794, -15.5804) knots 0 0 0 0 0 0 0.05 0.1 0.15 0.2 0.25 0.3 0.35 0.4 0.45 0.5 0.55 0.6 0.65 0.7 0.75 0.8 0.85 0.9 0.95 1 1 1 1 1 1
  line L81 (-20.4792, -16.3211) -> (-20.4792, -15.5211)
  line L82 (-36.2497, -24.0438) -> (-37.5084, -24.0463)
  circle A8 centre (42.6194, -14.6204) radius 0.3394
  line L83 (55.6595, -70.3446) -> (48.9725, -70.3446)
  line L84 (-17.2792, -16.7211) -> (-17.2792, -16.3211)
  line L85 (35.2994, -14.3804) -> (35.0594, -15.5804)
  line L86 (-19.9776, -16.2902) -> (-17.5602, -15.0775)
  spline S15 degree 2 poles (-36.2036, -19.5362) (-36.2582, -19.8553) (-36.2567, -20.5952) knots 0 0 0 1 1 1
  spline S16 degree 2 poles (-37.4162, -19.1857) (-37.315, -18.722) (-37.0414, -18.4025) knots 0 0 0 1 1 1
  line L87 (-20.4792, -16.7211) -> (-20.2167, -16.7211)
  spline S17 degree 2 poles (-26.8583, -20.9802) (-26.8605, -19.8703) (-27.3549, -19.3164) knots 0 0 0 1 1 1
  line L88 (43.5794, -26.8604) -> (42.8594, -24.2204)
  line L89 (58.1231, -71.5881) -> (64.8038, -71.5881)
  line L90 (-19.9792, -15.5211) -> (-19.9776, -16.2902)
  line L91 (-20.4792, -17.5348) -> (-20.4792, -16.6211)
  line L92 (-45.3709, -24.0622) -> (-47.2589, -24.066)
  arc A9 (49.8196, -60.0174) -> (48.5881, -59.6179) centre (49.2038, -59.8176) ccw
  line L93 (44.491, -23.8228) -> (45.3588, -26.8604)
  line L94 (-19.9792, -16.8211) -> (-19.9784, -17.1404)
  line L95 (-17.0167, -16.3211) -> (-17.0167, -15.5211)
  line L96 (-44.2611, -19.8076) -> (-45.3709, -24.0622)
  line L97 (-43.6528, -17.8248) -> (-42.4097, -22.7295)
  line L98 (-41.2377, -24.0538) -> (-43.1214, -24.0576)
  spline S18 degree 5 poles (45.3588, -26.8604) (45.3522, -26.8844) (45.3366, -26.931) (45.306, -26.9964) (45.251, -27.0747) (45.1583, -27.1574) (45.0419, -27.2243) (44.9034, -27.2748) (44.7464, -27.3084) (44.5771, -27.3249) (44.4031, -27.3243) (44.2324, -27.3066) (44.0726, -27.272) (43.9298, -27.221) (43.8075, -27.1541) (43.7073, -27.0719) (43.645, -26.9944) (43.6083, -26.9299) (43.5883, -26.8841) (43.5794, -26.8604) knots 0 0 0 0 0 0 0.066667 0.133333 0.2 0.266667 0.333333 0.4 0.466667 0.533333 0.6 0.666667 0.733333 0.8 0.866667 0.933333 1 1 1 1 1 1
  line L99 (-47.2589, -24.066) -> (-47.2715, -17.8321)
  line L100 (-17.2792, -16.3211) -> (-17.0167, -16.3211)
  line L101 (33.9794, -15.5804) -> (34.1976, -14.3804)
  line L102 (-43.1214, -24.0576) -> (-44.2611, -19.8076)
  line L103 (-38.7969, -24.0489) -> (-40.0555, -24.0514)
  line L104 (43.5442, -14.4114) -> (44.5818, -14.4546)
  line L105 (45.836, -66.4886) -> (43.4662, -59.2854)
  line L106 (40.6992, -15.9783) -> (40.2761, -16.3143)
  line L107 (60.5282, -19.2649) -> (61.8287, -14.4338)
  line L108 (-44.8647, -17.8273) -> (-43.6528, -17.8248)
  line L109 (-17.0167, -17.9211) -> (-20.4792, -17.9211)
  line L110 (41.2766, -66.5435) -> (41.2766, -59.5046)
  line L111 (61.3394, -20.1404) -> (60.5282, -19.2649)
  line L112 (60.1394, -14.4338) -> (59.0688, -18.6332)
  spline S19 degree 5 poles (59.0688, -18.6332) (59.0262, -18.6701) (58.9404, -18.7397) (58.81, -18.8309) (58.6326, -18.9261) (58.4045, -18.9982) (58.1695, -19.0194) (57.9273, -18.9862) (57.6777, -18.8979) (57.4211, -18.7575) (57.1582, -18.5696) (56.9432, -18.3846) (56.7795, -18.2276) (56.6693, -18.115) (56.6139, -18.0567) knots 0 0 0 0 0 0 0.1 0.2 0.3 0.4 0.5 0.6 0.7 0.8 0.9 1 1 1 1 1 1
  spline S20 degree 5 poles (36.8594, -16.5404) (36.846, -16.5465) (36.8186, -16.5585) (36.7753, -16.576) (36.7132, -16.598) (36.6281, -16.6233) (36.5356, -16.6461) (36.436, -16.6656) (36.3302, -16.6805) (36.2198, -16.6893) (36.1067, -16.6899) (35.9927, -16.6805) (35.8798, -16.6592) (35.7693, -16.625) (35.6621, -16.5774) (35.5586, -16.5165) (35.4789, -16.4573) (35.4208, -16.4071) (35.3828, -16.3711) (35.364, -16.3525) knots 0 0 0 0 0 0 0.066667 0.133333 0.2 0.266667 0.333333 0.4 0.466667 0.533333 0.6 0.666667 0.733333 0.8 0.866667 0.933333 1 1 1 1 1 1
  arc A10 (45.6038, -60.4176) -> (45.6038, -61.9232) centre (45.6038, -61.1704) ccw
  line L113 (-17.0167, -17.5348) -> (-17.0167, -16.7211)
  line L114 (-17.5602, -16.3775) -> (-17.5602, -15.6077)
  line L115 (-17.0167, -16.7211) -> (-17.2792, -16.7211)
  spline S21 degree 5 poles (36.7044, -15.7841) (36.6982, -15.7971) (36.6848, -15.8224) (36.6619, -15.8582) (36.6255, -15.9016) (36.5702, -15.9486) (36.5053, -15.9878) (36.4314, -16.0186) (36.3503, -16.0402) (36.2646, -16.0518) (36.178, -16.0524) (36.094, -16.0411) (36.0161, -16.0171) (35.9469, -15.9799) (35.888, -15.9297) (35.8399, -15.8666) (35.8103, -15.8062) (35.793, -15.7554) (35.7835, -15.7192) (35.7794, -15.7004) knots 0 0 0 0 0 0 0.066667 0.133333 0.2 0.266667 0.333333 0.4 0.466667 0.533333 0.6 0.666667 0.733333 0.8 0.866667 0.933333 1 1 1 1 1 1
  line L116 (48.5881, -59.6179) -> (45.7289, -68.432)
  line L117 (45.6194, -23.5004) -> (44.491, -23.8228)
  line L118 (-46.0922, -22.7369) -> (-44.8647, -17.8273)
  line L119 (55.6595, -70.9781) -> (48.9725, -70.9781) construction
  spline S22 degree 2 poles (-34.2379, -19.0071) (-34.5424, -18.776) (-35.0697, -18.777) knots 0 0 0 1 1 1
  line L120 (-32.5442, -20.711) -> (-32.5375, -24.0363)
  spline S23 degree 5 poles (49.078, -17.2) (49.0842, -17.1642) (49.0953, -17.0916) (49.1084, -16.9792) (49.1185, -16.8225) (49.1185, -16.615) (49.1052, -16.3966) (49.0774, -16.169) (49.0339, -15.9357) (48.9733, -15.702) (48.8941, -15.4746) (48.7946, -15.2604) (48.6738, -15.0659) (48.5307, -14.8958) (48.3656, -14.7529) (48.1789, -14.6379) (48.0127, -14.5682) (47.8788, -14.5283) (47.7855, -14.5071) (47.7378, -14.4979) knots 0 0 0 0 0 0 0.066667 0.133333 0.2 0.266667 0.333333 0.4 0.466667 0.533333 0.6 0.666667 0.733333 0.8 0.866667 0.933333 1 1 1 1 1 1
  spline S24 degree 2 poles (-33.7554, -17.9048) (-33.2936, -18.1101) (-33.025, -18.4391) knots 0 0 0 1 1 1
  spline S25 degree 5 poles (45.922, -17.1567) (45.9282, -17.121) (45.9393, -17.0484) (45.9524, -16.936) (45.9625, -16.7793) (45.9625, -16.5718) (45.9491, -16.3534) (45.9214, -16.1258) (45.8779, -15.8924) (45.8173, -15.6588) (45.738, -15.4314) (45.6386, -15.2172) (45.5177, -15.0226) (45.3747, -14.8526) (45.2096, -14.7097) (45.0228, -14.5947) (44.8566, -14.525) (44.7228, -14.485) (44.6294, -14.4639) (44.5818, -14.4546) knots 0 0 0 0 0 0 0.066667 0.133333 0.2 0.266667 0.333333 0.4 0.466667 0.533333 0.6 0.666667 0.733333 0.8 0.866667 0.933333 1 1 1 1 1 1
  line L121 (54.5831, -67.39) -> (51.2545, -65.4343)
  arc A11 (55.6595, -71.6116) -> (55.6595, -70.3446) centre (55.6595, -70.9781) ccw
  line L122 (50.0796, -20.5005) -> (49.7134, -21.7371)
  line L123 (46.5794, -26.8604) -> (45.6194, -23.5004)
  line L124 (-17.2792, -15.5211) -> (-17.2792, -15.1211)
  arc A12 (64.8038, -71.5881) -> (64.8038, -70.4149) centre (64.8038, -71.0015) ccw
  line L125 (-17.2792, -14.0211) -> (-17.8792, -13.4211)
  arc A13 (51.6038, -59.0823) -> (51.6038, -60.2085) centre (51.6038, -59.6454) ccw
  spline S26 degree 5 poles (46.2194, -27.4604) (46.2068, -27.4965) (46.1798, -27.5674) (46.1338, -27.6704) (46.0613, -27.8011) (45.9518, -27.9527) (45.8231, -28.092) (45.6749, -28.2176) (45.5072, -28.3273) (45.32, -28.4186) (45.1142, -28.4885) (44.8912, -28.5344) (44.6536, -28.5545) (44.4051, -28.5481) (44.1508, -28.516) (43.8963, -28.4599) (43.6472, -28.3817) (43.4086, -28.2836) (43.1842, -28.1675) (42.9763, -28.0349) (42.7861, -27.8868) (42.6484, -27.7565) (42.5532, -27.6522) (42.4934, -27.5798) (42.4644, -27.5429) knots 0 0 0 0 0 0 0.05 0.1 0.15 0.2 0.25 0.3 0.35 0.4 0.45 0.5 0.55 0.6 0.65 0.7 0.75 0.8 0.85 0.9 0.95 1 1 1 1 1 1
  line L126 (58.1231, -71.0015) -> (64.8038, -71.0015) construction
  spline S27 degree 2 poles (-35.0697, -18.777) (-35.6055, -18.7781) (-35.8772, -18.9976) knots 0 0 0 1 1 1
  spline S28 degree 2 poles (-30.0581, -22.071) (-29.9254, -22.5299) (-29.5612, -22.795) knots 0 0 0 1 1 1
  spline S29 degree 2 poles (-27.3421, -22.5332) (-26.8562, -22.0092) (-26.8583, -20.9802) knots 0 0 0 1 1 1
  spline S30 degree 2 poles (-30.2513, -17.9827) (-29.5014, -17.69) (-28.7317, -17.6884) knots 0 0 0 1 1 1
  spline S31 degree 5 poles (47.2994, -26.8604) (47.2908, -26.8866) (47.2724, -26.9377) (47.2414, -27.0105) (47.1931, -27.1001) (47.1203, -27.1985) (47.034, -27.2822) (46.9332, -27.3501) (46.8174, -27.4016) (46.6873, -27.4375) (46.5441, -27.459) (46.4198, -27.4657) (46.3215, -27.4652) (46.2538, -27.4624) (46.2194, -27.4604) knots 0 0 0 0 0 0 0.1 0.2 0.3 0.4 0.5 0.6 0.7 0.8 0.9 1 1 1 1 1 1
  arc A14 (59.7448, -67.7352) -> (60.2628, -68.7001) centre (60.0038, -68.2176) ccw
  spline S32 degree 2 poles (-30.4653, -23.6515) (-31.119, -23.1659) (-31.3078, -22.3074) knots 0 0 0 1 1 1
  line L127 (56.2718, -74.8176) -> (56.2718, -77.2176)
  spline S33 degree 2 poles (-33.025, -18.4391) (-32.7565, -18.7681) (-32.6707, -19.1294) knots 0 0 0 1 1 1
  spline S34 degree 2 poles (-27.0257, -18.0953) (-26.2977, -18.5042) (-25.9305, -19.2667) knots 0 0 0 1 1 1
  spline S35 degree 2 poles (-29.5612, -22.795) (-29.1971, -23.06) (-28.6528, -23.0589) knots 0 0 0 1 1 1
  line L128 (54.1966, -68.0478) -> (50.868, -66.0921) construction
  line L129 (45.8889, -22.4312) -> (47.4568, -16.9406)
  line L130 (57.0038, -59.6454) -> (51.6038, -59.6454) construction
  line L131 (-17.2792, -15.1211) -> (-17.0167, -15.1211)
  line L132 (-33.7962, -24.0388) -> (-33.803, -20.6625)
  line L133 (-30.1216, -20.0895) -> (-28.6801, -20.0866)
  line L134 (57.5739, -68.8176) -> (57.5739, -61.8275)
  spline S36 degree 5 poles (52.5226, -22.8607) (52.5269, -22.8164) (52.5329, -22.7275) (52.5341, -22.5931) (52.5198, -22.412) (52.4747, -22.1827) (52.4019, -21.9514) (52.3008, -21.7202) (52.172, -21.4928) (52.0169, -21.2747) (51.8375, -21.0724) (51.6364, -20.8925) (51.4159, -20.741) (51.1781, -20.6221) (50.9248, -20.5378) (50.6573, -20.4884) (50.4326, -20.4763) (50.2583, -20.4825) (50.1396, -20.4934) (50.0796, -20.5005) knots 0 0 0 0 0 0 0.066667 0.133333 0.2 0.266667 0.333333 0.4 0.466667 0.533333 0.6 0.666667 0.733333 0.8 0.866667 0.933333 1 1 1 1 1 1
  line L135 (-20.2167, -15.5211) -> (-20.2167, -15.1211)
  arc A15 (56.2718, -77.2176) -> (57.7359, -77.2176) centre (57.0038, -77.2176) ccw
  line L136 (-20.4792, -15.5211) -> (-20.2167, -15.5211)
  line L137 (-20.4792, -15.1211) -> (-20.4792, -14.2211)
  line L138 (-30.1232, -19.2986) -> (-30.1216, -20.0895)
  line L139 (-20.2167, -15.1211) -> (-20.4792, -15.1211)
  line L140 (46.7002, -14.4546) -> (47.7378, -14.4979)
  line L141 (-18.5375, -12.7629) -> (-18.9584, -12.7629)
  spline S37 degree 2 poles (-27.3549, -19.3164) (-27.8493, -18.7625) (-28.6488, -18.7641) knots 0 0 0 1 1 1
  line L142 (50.3326, -25.0449) -> (50.9366, -22.8645)
  line L143 (47.2994, -26.8604) -> (46.5794, -26.8604)
  line L144 (-17.9792, -13.3211) -> (-18.3792, -12.9211)
  line L145 (57.7359, -77.2176) -> (57.7359, -74.8176)
  line L146 (-17.8792, -13.4211) -> (-19.6167, -13.4211)
  line L147 (60.2628, -68.7001) -> (64.0367, -66.674)
  line L148 (-17.5602, -14.3077) -> (-19.9792, -15.5211)
  line L149 (-17.5602, -15.0775) -> (-17.5602, -14.3077)
  line L150 (63.5187, -65.7092) -> (59.7448, -67.7352)
  line L151 (-18.6809, -12.6194) -> (-18.8149, -12.6194)
  line L152 (-17.9792, -13.3211) -> (-19.5167, -13.3211)
  line L153 (57.0038, -77.2176) -> (57.0038, -74.8176) construction
  spline S38 degree 2 poles (-25.9305, -19.2667) (-25.5633, -20.0293) (-25.5615, -20.9265) knots 0 0 0 1 1 1
  line L154 (-28.6801, -20.0866) -> (-28.678, -21.1369)
  spline S39 degree 2 poles (-28.6488, -18.7641) (-29.0442, -18.7649) (-29.4415, -18.9209) knots 0 0 0 1 1 1
  line L155 (-20.2167, -14.0211) -> (-19.6167, -13.4211)
  spline S40 degree 2 poles (-33.803, -20.6625) (-33.8046, -19.8588) (-33.8519, -19.6208) knots 0 0 0 1 1 1
  line L156 (48.793, -25.0449) -> (50.3326, -25.0449)
  line L157 (-18.3792, -12.9211) -> (-19.1167, -12.9211)
  spline S41 degree 2 poles (-32.6707, -19.1294) (-32.5463, -19.6649) (-32.5442, -20.711) knots 0 0 0 1 1 1
  spline S42 degree 5 poles (47.4568, -16.9406) (47.4733, -16.9063) (47.5032, -16.8386) (47.5382, -16.7394) (47.565, -16.6123) (47.5632, -16.4623) (47.5231, -16.3219) (47.4422, -16.1919) (47.3196, -16.0723) (47.158, -15.9626) (46.9606, -15.862) (46.7765, -15.7881) (46.6247, -15.7361) (46.5175, -15.703) (46.4624, -15.6868) knots 0 0 0 0 0 0 0.1 0.2 0.3 0.4 0.5 0.6 0.7 0.8 0.9 1 1 1 1 1 1
  arc A16 (51.2545, -65.4343) -> (50.4816, -66.7499) centre (50.868, -66.0921) ccw
  arc A17 (57.7359, -74.8176) -> (56.2718, -74.8176) centre (57.0038, -74.8176) ccw
  line L158 (47.7162, -22.4312) -> (45.8889, -22.4312)
  line L159 (-19.5167, -13.3211) -> (-19.1167, -12.9211)
  line L160 (46.4624, -15.6868) -> (46.7002, -14.4546)
  spline S43 degree 2 poles (-27.1587, -23.8213) (-27.7577, -24.1329) (-28.6507, -24.1347) knots 0 0 0 1 1 1
  line L161 (-17.0167, -14.2211) -> (-17.2792, -14.2211)